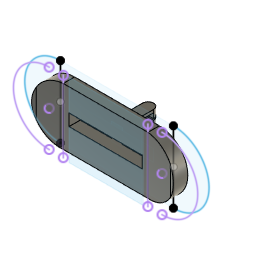
Skater v2 (Autodesk Fusion 360 design; units mm, degrees)
Autodesk Fusion 360 part; units mm, degrees
sketch "Sketch1" plane through (0, 0, 0) normal (0, 0, 1) x (1, 0, 0)
  circle A0 centre (2.87141, -3.259439) radius 3.9
  line L0 (2.87141, -3.259439) -> (6.77141, -3.259439)
  line L1 (6.77141, -3.259439) -> (-1.02859, -3.259439)
  dimension "d1" = 7.8
  constraint horizontal L0
  constraint parallel L0 L1
  measures "d1" diameter of A0
extrude "Extrude1" add sketch "Sketch1" along normal blind 3.7 contours A0 L0 L1 picked at (0.844332, -1.642898) makes body 1
sketch "Sketch2" plane through (0, 0, 0) normal (0, 0, -1) x (1, 0, 0)
  arc A0 (-1.02859, 3.259439) -> (6.77141, 3.259439) centre (2.87141, 3.259439) ccw
  line L0 (6.77141, 3.259439) -> (-1.02859, 3.259439)
  line L1 (-1.02859, 3.259439) -> (6.77141, 3.259439)
  line L2 (6.77141, 3.259439) -> (6.77141, 25.259439)
  line L3 (6.77141, 25.259439) -> (-1.02859, 25.259439)
  line L4 (-1.02859, 25.259439) -> (-1.02859, 3.259439)
  dimension "d4" = 22
  constraint horizontal L1
  constraint vertical L2
  constraint horizontal L3
  constraint vertical L4
extrude "Extrude2" add sketch "Sketch2" along normal blind 2 contours A0 L0 L1 | L0 L1 L2 L3 L4 picked at (3.53593, 1.939851) picked at (1.57141, 17.926105) bodies 1
sketch "Sketch3" plane through (6.77141, 0, 0) normal (1, 0, 0) x (0, 1, 0)
  line L0 (-3.259439, 0) -> (-25.259439, 0)
  line L1 (-25.259439, 0) -> (-25.259439, -2)
  line L2 (-25.259439, -2) -> (-3.259439, -2)
  line L3 (-3.259439, -2) -> (-3.259439, 0)
  line L4 (-12.859448, 0) -> (-15.659448, 0)
  line L5 (-14.259439, -1) -> (-12.859448, 0)
  line L6 (-14.259439, -1) -> (-15.659448, 0)
extrude "Extrude3" cut sketch "Sketch3" against normal blind 15 contours L0 L4 L5 L6 picked at (-14.259445, -0.333333) bodies 1
copy_body "CopyPasteBodies1" bodies 1 makes body 2
move_body "Move1" bodies 2 to x (1, 0, 0) y (0, 1, 0) z (0, 0, 1) at (0, 0, 6)
move_body "Move2" bodies 2 to x (-1, 0, 0) y (0, 1, 0) z (0, 0, -1) at (5.74282, 0, 14.4)
sketch "Sketch7" plane through (0, -25.259439, 0) normal (0, -1, 0) x (1, 0, 0)
  line L0 (-1.02859, 8.4) -> (6.77141, 8.4)
  line L1 (6.77141, 8.4) -> (6.77141, 10.4)
  line L2 (6.77141, 10.4) -> (-1.02859, 10.4)
  line L3 (-1.02859, 10.4) -> (-1.02859, 8.4)
sketch "Sketch8" plane through (0, 0, 10.4) normal (0, 0, 1) x (-1, 0, 0)
  line L0 (-6.77141, 25.259439) -> (-6.77141, 3.259439)
  arc A0 (-6.77141, 3.259439) -> (1.02859, 3.259439) centre (-2.87141, 3.259439) ccw
  line L1 (1.02859, 3.259439) -> (1.02859, 25.259439)
  line L2 (1.02859, 25.259439) -> (-6.77141, 25.259439)
  line L3 (-6.77141, 25.259439) -> (1.02859, 25.259439)
  line L4 (1.02859, 25.259439) -> (1.02859, 33.259439)
  line L5 (1.02859, 33.259439) -> (-6.77141, 33.259439)
  line L6 (-6.77141, 33.259439) -> (-6.77141, 25.259439)
  dimension "d10" = 8
  constraint horizontal L3
  constraint vertical L4
  constraint horizontal L5
  constraint vertical L6
sketch "Sketch9" plane through (0, 0, -2) normal (0, 0, -1) x (1, 0, 0)
  line L0 (-1.02859, 25.259439) -> (-1.02859, 3.259439)
  arc A0 (-1.02859, 3.259439) -> (6.77141, 3.259439) centre (2.87141, 3.259439) ccw
  line L1 (6.77141, 3.259439) -> (6.77141, 25.259439)
  line L2 (6.77141, 25.259439) -> (-1.02859, 25.259439)
  line L3 (-1.02859, 25.259439) -> (6.77141, 25.259439)
  line L4 (6.77141, 25.259439) -> (6.77141, 33.259439)
  line L5 (6.77141, 33.259439) -> (-1.02859, 33.259439)
  line L6 (-1.02859, 33.259439) -> (-1.02859, 25.259439)
  dimension "d11" = 8
  constraint horizontal L3
  constraint vertical L4
  constraint horizontal L5
  constraint vertical L6
extrude "Extrude4" add sketch "Sketch9" along normal blind 5 separate body contours L2 L3 L4 L5 L6 picked at (1.57141, 30.592772) makes body 3
extrude "Extrude5" add sketch "Sketch8" along normal blind 5 separate body contours L2 L3 L4 L5 L6 picked at (-4.17141, 30.592772) makes body 4
extrude "Extrude6" add 1 faces at (1.57141, -30.592772, -2) along direction (0, 0, 1) blind 2 on bodies 3 bodies 3 1
extrude "Extrude7" add 1 faces at (4.17141, -30.592772, 10.4) along direction (0, 0, -1) blind 2 on bodies 4 bodies 4 2
sketch "Sketch10" plane through (-1.02859, 0, 0) normal (-1, 0, 0) x (0, -1, 0)
  line L0 (33.259439, 8.4) -> (33.259439, 15.4)
  line L1 (33.259439, 15.4) -> (25.259439, 15.4)
  line L2 (25.259439, 15.4) -> (25.259439, 10.4)
  line L3 (25.259439, 10.4) -> (3.259439, 10.4)
  line L4 (3.259439, 10.4) -> (3.259439, 8.4)
  line L5 (3.259439, 8.4) -> (12.859448, 8.4)
  line L6 (12.859448, 8.4) -> (14.259439, 9.4)
  line L7 (14.259439, 9.4) -> (15.659448, 8.4)
  line L8 (15.659448, 8.4) -> (33.259439, 8.4)
  line L9 (12.859448, 8.4) -> (15.659448, 8.4)
sketch "Sketch11" plane through (-1.02859, 0, 0) normal (-1, 0, 0) x (0, -1, 0)
  line L0 (25.259439, -2) -> (25.259439, -7)
  line L1 (25.259439, -7) -> (33.259439, -7)
  line L2 (33.259439, -7) -> (33.259439, 0)
  line L3 (33.259439, 0) -> (15.659448, 0)
  line L4 (15.659448, 0) -> (14.259439, -1)
  line L5 (14.259439, -1) -> (12.859448, 0)
  line L6 (12.859448, 0) -> (3.259439, 0)
  line L7 (3.259439, 0) -> (3.259439, -2)
  line L8 (3.259439, -2) -> (25.259439, -2)
  line L9 (15.659448, 0) -> (12.859448, 0)
extrude "Extrude8" add sketch "Sketch10" sketch "Sketch11" against normal blind 7.8 contours L6 L7 L9 picked at (14.259445, 8.733333) of sketch 2 contours L4 L5 L9 picked at (14.259445, -0.333333) bodies 3 4
sketch "Sketch12" plane through (-1.02859, 0, 0) normal (-1, 0, 0) x (0, -1, 0)
  line L0 (33.259439, 8.4) -> (33.259439, 15.4)
  line L1 (33.259439, 15.4) -> (25.259439, 15.4)
  line L2 (25.259439, 15.4) -> (25.259439, 10.4)
  line L3 (25.259439, 10.4) -> (3.259439, 10.4)
  line L4 (3.259439, 10.4) -> (3.259439, 8.4)
  line L5 (3.259439, 8.4) -> (33.259439, 8.4)
  line L6 (25.259439, 10.4) -> (14.259439, 10.4)
  line L7 (15.659854, 10.4) -> (12.859854, 10.4)
  line L8 (12.859854, 10.4) -> (14.259439, 9.4)
  line L9 (14.259439, 9.4) -> (15.659854, 10.4)
  dimension "d23" = 2.8
extrude "Extrude9" cut sketch "Sketch12" against normal blind 8 contours L3 L6 L7 L8 L9 picked at (14.726244, 10.066667) bodies 4
sketch "Sketch13" plane through (-1.02859, 0, 0) normal (-1, 0, 0) x (0, -1, 0)
  line L0 (25.259439, -2) -> (25.259439, -7)
  line L1 (25.259439, -7) -> (33.259439, -7)
  line L2 (33.259439, -7) -> (33.259439, 0)
  line L3 (33.259439, 0) -> (3.259439, 0)
  line L4 (3.259439, 0) -> (3.259439, -2)
  line L5 (3.259439, -2) -> (25.259439, -2)
  line L6 (12.859439, -2) -> (14.259439, -1)
  line L7 (14.259439, -1) -> (15.659439, -2)
extrude "Extrude10" cut sketch "Sketch13" against normal blind 8 contours L5 L6 L7 picked at (14.259439, -1.666667) bodies 3
extrude "Extrude11" add 1 faces at (4.17141, -30.592772, 15.4) along direction (0, 0, 1) blind 15 on bodies 4 bodies 4
extrude "Extrude12" add 1 faces at (1.57141, -30.592772, -7) along direction (0, 0, -1) blind 15 on bodies 3 bodies 3
sketch "Sketch14" plane through (6.77141, 0, 0) normal (1, 0, 0) x (0, 1, 0)
  line L0 (-15.659439, -2) -> (-14.259439, -1)
  line L1 (-14.259439, -1) -> (-12.859439, -2)
  line L2 (-12.859439, -2) -> (-3.259439, -2)
  line L3 (-3.259439, -2) -> (-3.259439, 0)
  line L4 (-3.259439, 0) -> (-33.259439, 0)
  line L5 (-33.259439, 0) -> (-33.259439, -22)
  line L6 (-33.259439, -22) -> (-25.259439, -22)
  line L7 (-25.259439, -22) -> (-25.259439, -2)
  line L8 (-25.259439, -2) -> (-15.659439, -2)
  line L9 (-25.259439, -2) -> (-25.259439, 0)
  constraint perpendicular L4 L9
sketch "Sketch15" plane through (6.77141, 0, 0) normal (1, 0, 0) x (0, 1, 0)
  line L0 (-12.859854, 10.4) -> (-14.259439, 9.4)
  line L1 (-14.259439, 9.4) -> (-15.659854, 10.4)
  line L2 (-15.659854, 10.4) -> (-25.259439, 10.4)
  line L3 (-25.259439, 10.4) -> (-25.259439, 30.4)
  line L4 (-25.259439, 30.4) -> (-33.259439, 30.4)
  line L5 (-33.259439, 30.4) -> (-33.259439, 8.4)
  line L6 (-33.259439, 8.4) -> (-3.259439, 8.4)
  line L7 (-3.259439, 8.4) -> (-3.259439, 10.4)
  line L8 (-3.259439, 10.4) -> (-12.859854, 10.4)
  line L9 (-25.259439, 10.4) -> (-25.259439, 8.4)
  constraint perpendicular L6 L9
sketch "Sketch16" plane through (-1.02859, 0, 0) normal (-1, 0, 0) x (0, -1, 0)
  line L0 (15.659854, 10.4) -> (14.259439, 9.4)
  line L1 (14.259439, 9.4) -> (12.859854, 10.4)
  line L2 (12.859854, 10.4) -> (3.259439, 10.4)
  line L3 (3.259439, 10.4) -> (3.259439, 8.4)
  line L4 (3.259439, 8.4) -> (33.259439, 8.4)
  line L5 (33.259439, 8.4) -> (33.259439, 30.4)
  line L6 (33.259439, 30.4) -> (25.259439, 30.4)
  line L7 (25.259439, 30.4) -> (25.259439, 10.4)
  line L8 (25.259439, 10.4) -> (15.659854, 10.4)
  line L9 (25.259439, 10.4) -> (25.259439, 8.4)
  constraint perpendicular L4 L9
sketch "Sketch17" plane through (-1.02859, 0, 0) normal (-1, 0, 0) x (0, -1, 0)
  line L0 (14.259439, -1) -> (15.659439, -2)
  line L1 (15.659439, -2) -> (25.259439, -2)
  line L2 (25.259439, -2) -> (25.259439, -22)
  line L3 (25.259439, -22) -> (33.259439, -22)
  line L4 (33.259439, -22) -> (33.259439, 0)
  line L5 (33.259439, 0) -> (3.259439, 0)
  line L6 (3.259439, 0) -> (3.259439, -2)
  line L7 (3.259439, -2) -> (12.859439, -2)
  line L8 (12.859439, -2) -> (14.259439, -1)
  line L9 (25.259439, -2) -> (25.259439, 0)
  constraint perpendicular L5 L9
extrude "Extrude13" add sketch "Sketch17" sketch "Sketch16" along normal blind 7 contours L2 L3 L4 L5 L9 picked at (30.592772, -8) of sketch 2 contours L4 L5 L6 L7 L9 picked at (30.592772, 16.4) bodies 3 4
extrude "Extrude14" add sketch "Sketch15" sketch "Sketch14" along normal blind 7 contours L3 L4 L5 L6 L9 picked at (-30.592772, 16.4) of sketch 2 contours L4 L5 L6 L7 L9 picked at (-30.592772, -8) bodies 3 4
extrude "Extrude15" add 2 faces at (-8.02859, -30.592772, 23.066667) (-8.02859, -27.926105, -7.333333) along direction (-1, 0, 0) blind 15 on bodies 3 4 bodies 4 3
extrude "Extrude16" add 2 faces at (13.77141, -27.926105, 15.733333) (13.77141, -27.926105, -14.666667) along direction (1, 0, 0) blind 15 on bodies 3 4 bodies 4 3
sketch "Sketch18" plane through (0, -33.259439, 0) normal (0, -1, 0) x (1, 0, 0)
  line L0 (-23.02859, -22) -> (28.77141, -22)
  line L1 (28.77141, -22) -> (28.77141, 0)
  line L2 (28.77141, 0) -> (-23.02859, 0)
  line L3 (-23.02859, 0) -> (-23.02859, -22)
sketch "Sketch19" plane through (0, -33.259439, 0) normal (0, -1, 0) x (1, 0, 0)
  line L0 (28.77141, 30.4) -> (-23.02859, 30.4)
  line L1 (-23.02859, 30.4) -> (-23.02859, 8.4)
  line L2 (-23.02859, 8.4) -> (28.77141, 8.4)
  line L3 (28.77141, 8.4) -> (28.77141, 30.4)
sketch "Sketch20" plane through (28.77141, 0, 0) normal (1, 0, 0) x (0, 1, 0)
  line L0 (-25.259439, 30.4) -> (-33.259439, 30.4)
  line L1 (-33.259439, 30.4) -> (-33.259439, 8.4)
  line L2 (-33.259439, 8.4) -> (-25.259439, 8.4)
  line L3 (-25.259439, 8.4) -> (-25.259439, 30.4)
  line L4 (-33.259439, 30.4) -> (-25.259439, 30.4)
  line L5 (-25.259439, 30.4) -> (-25.259439, 1.557933)
  line L6 (-25.259439, 1.557933) -> (-33.259439, 1.557933)
  line L7 (-33.259439, 1.557933) -> (-33.259439, 30.4)
  constraint horizontal L4
  constraint vertical L5
  constraint horizontal L6
  constraint vertical L7
sketch "Sketch21" plane through (28.77141, 0, 0) normal (1, 0, 0) x (0, 1, 0)
  line L0 (-25.259439, -22) -> (-25.259439, 0)
  line L1 (-25.259439, 0) -> (-33.259439, 0)
  line L2 (-33.259439, 0) -> (-33.259439, -22)
  line L3 (-33.259439, -22) -> (-25.259439, -22)
  line L4 (-25.259439, -22) -> (-33.259439, -22)
  line L5 (-33.259439, -22) -> (-33.259439, 7.010698)
  line L6 (-33.259439, 7.010698) -> (-25.259439, 7.010698)
  line L7 (-25.259439, 7.010698) -> (-25.259439, -22)
  constraint horizontal L4
  constraint vertical L5
  constraint horizontal L6
  constraint vertical L7
extrude "Extrude17" add sketch "Sketch20" sketch "Sketch21" along normal blind 1 contours L0 L1 L2 L3 L4 L5 L7 | L2 L5 L6 L7 picked at (-27.926105, 15.733333) picked at (-30.592772, 6.119311) of sketch 2 contours L0 L1 L2 L3 L4 L5 L7 | L1 L5 L6 L7 picked at (-27.926105, -14.666667) picked at (-30.592772, 4.673798) bodies 3 4
sketch "Sketch22" plane through (0, -33.259439, 0) normal (0, -1, 0) x (1, 0, 0)
sketch "Sketch23" plane through (2.87141, -33.259439, -11) normal (0, -1, 0) x (1, 0, 0)
sketch "Sketch24" plane through (0, -33.259439, 0) normal (0, -1, 0) x (1, 0, 0)
sketch "Sketch25" plane through (0, -33.259439, 0) normal (0, -1, 0) x (1, 0, 0)
  line L0 (-23.02859, -22) -> (29.77141, -22)
  line L1 (29.77141, -22) -> (29.77141, 30.4)
  line L2 (29.77141, 30.4) -> (-23.02859, 30.4)
  line L3 (-23.02859, 30.4) -> (-23.02859, 8.4)
  line L4 (-23.02859, 8.4) -> (28.77141, 8.4)
  line L5 (28.77141, 8.4) -> (28.77141, 0)
  line L6 (28.77141, 0) -> (-23.02859, 0)
  line L7 (-23.02859, 0) -> (-23.02859, -22)
extrude "Extrude18" add 1 faces at (29.77141, -30.592772, 12.933333) along direction (1, 0, 0) blind 13 on bodies 3 bodies 3
sketch "Sketch26" plane through (-23.02859, 0, 0) normal (-1, 0, 0) x (0, -1, 0)
  line L0 (25.259439, 30.4) -> (25.259439, 8.4)
  line L1 (25.259439, 8.4) -> (33.259439, 8.4)
  line L2 (33.259439, 8.4) -> (33.259439, 30.4)
  line L3 (33.259439, 30.4) -> (25.259439, 30.4)
  line L4 (25.259439, 30.4) -> (33.259439, 30.4)
  line L5 (33.259439, 30.4) -> (33.259439, -16.961033)
  line L6 (33.259439, -16.961033) -> (25.259439, -16.961033)
  line L7 (25.259439, -16.961033) -> (25.259439, 30.4)
  constraint horizontal L4
  constraint vertical L5
  constraint horizontal L6
  constraint vertical L7
sketch "Sketch27" plane through (-23.02859, 0, 0) normal (-1, 0, 0) x (0, -1, 0)
  line L0 (25.259439, -22) -> (33.259439, -22)
  line L1 (33.259439, -22) -> (33.259439, 0)
  line L2 (33.259439, 0) -> (25.259439, 0)
  line L3 (25.259439, 0) -> (25.259439, -22)
  line L4 (33.259439, -22) -> (25.259439, -22)
  line L5 (25.259439, -22) -> (25.259439, -5.279262)
  line L6 (25.259439, -5.279262) -> (33.259439, -5.279262)
  line L7 (33.259439, -5.279262) -> (33.259439, -22)
  constraint horizontal L4
  constraint vertical L5
  constraint horizontal L6
  constraint vertical L7
extrude "Extrude19" add sketch "Sketch26" sketch "Sketch27" along normal blind 14 contours L0 L1 L2 L3 L4 L5 L7 | L1 L5 L6 L7 picked at (27.926105, 23.066667) picked at (30.592772, -8.507356) of sketch 2 contours L0 L1 L3 L4 L5 L6 L7 picked at (27.926105, -10.852841) bodies 3
sketch "Sketch28" plane through (0, -33.259439, 0) normal (0, -1, 0) x (1, 0, 0)
  line L0 (-23.02859, 8.4) -> (28.77141, 8.4)
  line L1 (28.77141, 8.4) -> (28.77141, 0)
  line L2 (28.77141, 0) -> (-23.02859, 0)
  line L3 (-23.02859, 0) -> (-23.02859, 8.4)
  line L4 (42.77141, 30.4) -> (-37.02859, 30.4)
  line L5 (-37.02859, 30.4) -> (-37.02859, -22)
  line L6 (-37.02859, -22) -> (42.77141, -22)
  line L7 (42.77141, -22) -> (42.77141, 30.4)
  arc A0 (-37.02859, 30.4) -> (-37.02859, -22) centre (-37.02859, 4.2) ccw
  arc A1 (42.77141, -22) -> (42.77141, 30.4) centre (42.77141, 4.2) ccw
  constraint tangent L6 A0
  constraint tangent L4 A0
  constraint tangent L6 A1
  constraint tangent L4 A1
extrude "Extrude20" add sketch "Sketch28" against normal blind 8 contours L7 A1 | L5 A0 picked at (51.480323, 4.852643) picked at (-45.737503, 3.547357) bodies 3
extrude "Extrude21" add 1 faces at (11.504743, -33.259439, -14.666667) along direction (0, -1, 0) blind 5 thin wall 1 inside on bodies 3 bodies 3
sketch "Sketch29" plane through (0, -33.259439, 0) normal (0, -1, 0) x (1, 0, 0)
  line L0 (-24.02859, -1) -> (-24.02859, 9.4)
  line L1 (-24.02859, 9.4) -> (29.77141, 9.4)
  line L2 (29.77141, 9.4) -> (29.77141, -1)
  line L3 (29.77141, -1) -> (-24.02859, -1)
  line L4 (42.77141, 29.4) -> (-37.02859, 29.4)
  arc A0 (-37.02859, 29.4) -> (-37.02859, -21) centre (-37.02859, 4.2) ccw
  line L5 (-37.02859, -21) -> (42.77141, -21)
  arc A1 (42.77141, -21) -> (42.77141, 29.4) centre (42.77141, 4.2) ccw
  line L6 (-37.02859, 29.4) -> (-27.02859, 29.4)
  line L7 (42.77141, 29.4) -> (32.77141, 29.4)
  line L8 (32.77141, 29.4) -> (32.77141, -21)
  line L9 (-27.02859, 29.4) -> (-27.02859, -21)
  dimension "d55" = 10
  dimension "d56" = 10
  constraint perpendicular L0 L6
  constraint parallel L4 L7
  constraint perpendicular L5 L8
  constraint perpendicular L5 L9
sketch "Sketch30" plane through (0, -33.259439, 0) normal (0, -1, 0) x (1, 0, 0)
sketch "Sketch31" plane through (0, -33.259439, 0) normal (0, -1, 0) x (1, 0, 0)
sketch "Sketch32" plane through (0, -33.259439, 0) normal (0, -1, 0) x (1, 0, 0)
sketch "Sketch33" plane through (0, 0, 0) normal (0, 1, 0) x (1, 0, 0)
sketch "Sketch35" plane through (-44.62859, -33.259439, 4.2) normal (0, -1, 0) x (1, 0, 0)
  line L0 (17.6, 25.2) -> (17.6, -25.2)
  arc A0 (7.6, 25.2) -> (7.6, -25.2) centre (7.6, 0) ccw
  line L1 (77.4, 25.2) -> (77.4, -25.2)
  arc A1 (87.4, -25.2) -> (87.4, 25.2) centre (87.4, 0) ccw
revolve "Revolve1" add sketch "Sketch29" angle 5 about axis through (-27.02859, -33.259439, 29.4) along (0, 0, 1) contours L4 A0 L5 L6 L9 picked at (-42.742041, -1.957636) bodies 3
sketch "Sketch36" plane through (0, -33.259439, 0) normal (0, -1, 0) x (1, 0, 0)
  line L0 (-27.02859, 29.4) -> (-27.02859, -21)
  line L1 (-27.02859, -21) -> (42.77141, -21)
  arc A0 (42.77141, -21) -> (42.77141, 29.4) centre (42.77141, 4.2) ccw
  line L2 (42.77141, 29.4) -> (-27.02859, 29.4)
  line L3 (-24.02859, -1) -> (-24.02859, 9.4)
  line L4 (-24.02859, 9.4) -> (29.77141, 9.4)
  line L5 (29.77141, 9.4) -> (29.77141, -1)
  line L6 (29.77141, -1) -> (-24.02859, -1)
  line L7 (32.77141, 29.4) -> (32.77141, -21)
  point P0 (32.77141, 29.4)
  point P1 (32.77141, -21)
revolve "Revolve2" add sketch "Sketch36" angle 5 about axis through (32.77141, -33.259439, 29.4) along (0, 0, -1) contours L1 A0 L2 L7 picked at (54.605428, 5.237314) bodies 3
sketch "Sketch37" plane through (-2.638785, -30.161448, 0) normal (-0.087156, -0.996195, 0) x (0.996195, -0.087156, 0)
  line L0 (35.545456, 29.4) -> (35.545456, -21)
  line L1 (35.545456, -21) -> (45.545456, -21)
  arc A0 (45.545456, -21) -> (45.545456, 29.4) centre (45.545456, 4.2) ccw
  line L2 (45.545456, 29.4) -> (35.545456, 29.4)
  line L3 (53.145456, -19.826652) -> (53.145456, 28.226652)
sketch "Sketch38" plane through (2.682408, -30.660063, 0) normal (0.087156, -0.996195, 0) x (0.996195, 0.087156, 0)
  arc A0 (-39.824489, 29.4) -> (-39.824489, -21) centre (-39.824489, 4.2) ccw
  line L0 (-39.824489, -21) -> (-29.824489, -21)
  line L1 (-29.824489, -21) -> (-29.824489, 29.4)
  line L2 (-29.824489, 29.4) -> (-39.824489, 29.4)
  line L3 (-47.424489, 28.226652) -> (-47.424489, -19.826652)
revolve "Revolve3" add sketch "Sketch37" angle 10 about axis through (50.304437, -34.79338, -19.826652) along (0, 0, -1) contours A0 L3 picked at (57.899083, 0.021459) bodies 3
revolve "Revolve4" add sketch "Sketch38" angle 10 about axis through (-44.561617, -34.79338, 28.226652) along (0, 0, 1) contours A0 L3 picked at (-56.476506, 1.698018) bodies 3
sketch "Sketch39" plane through (-5.328587, -19.886556, 0) normal (-0.258819, -0.965926, 0) x (0.965926, -0.258819, 0)
  arc A0 (57.595544, -19.826652) -> (57.595544, 28.226652) centre (49.995544, 4.2) ccw
  line L0 (57.595544, 28.226652) -> (57.595544, -19.826652)
  line L1 (66.395544, -14.933217) -> (66.395544, 23.333217)
sketch "Sketch40" plane through (5.713283, -21.322261, 0) normal (0.258819, -0.965926, 0) x (0.965926, 0.258819, 0)
  arc A0 (-52.048406, 28.226652) -> (-52.048406, -19.826652) centre (-44.448406, 4.2) ccw
  line L0 (-52.048406, -19.826652) -> (-52.048406, 28.226652)
  line L1 (-60.848406, -14.933217) -> (-60.848406, 23.333217)
revolve "Revolve5" add sketch "Sketch40" angle 10 about axis through (-53.061764, -37.070987, -14.933217) along (0, 0, 1) contours A0 L1 picked at (-64.55212, 2.148555) bodies 3
revolve "Revolve6" add sketch "Sketch39" angle 10 about axis through (58.804584, -37.070987, -14.933217) along (0, 0, -1) contours A0 L1 picked at (67.979106, 8.766647) bodies 3
extrude "Extrude22" cut 1 faces at (-10.42859, -38.259439, -21.333333) along direction (0, 1, 0) blind 20 on bodies 3 bodies 3
extrude "Extrude23" cut 1 faces at (-5.761923, -38.259439, -0.666667) along direction (0, 1, 0) blind 5 on bodies 3 bodies 3
sketch "Sketch41" plane through (0, -25.259439, 0) normal (0, 1, 0) x (-1, 0, 0)
  line L0 (-42.77141, -21) -> (37.02859, -21)
  arc A0 (37.02859, -21) -> (37.02859, 29.4) centre (37.02859, 4.2) ccw
  line L1 (37.02859, 29.4) -> (-42.77141, 29.4)
  arc A1 (-42.77141, 29.4) -> (-42.77141, -21) centre (-42.77141, 4.2) ccw
  line L2 (23.02859, 8.4) -> (23.02859, 0)
  line L3 (23.02859, 0) -> (1.02859, 0)
  line L4 (1.02859, 0) -> (1.02859, -2)
  line L5 (1.02859, -2) -> (-6.77141, -2)
  line L6 (-6.77141, -2) -> (-6.77141, 0)
  line L7 (-6.77141, 0) -> (-28.77141, 0)
  line L8 (-28.77141, 0) -> (-28.77141, 8.4)
  line L9 (-28.77141, 8.4) -> (-6.77141, 8.4)
  line L10 (-6.77141, 8.4) -> (-6.77141, 10.4)
  line L11 (-6.77141, 10.4) -> (1.02859, 10.4)
  line L12 (1.02859, 10.4) -> (1.02859, 8.4)
  line L13 (1.02859, 8.4) -> (23.02859, 8.4)
  line L14 (-42.77141, 29.4) -> (-42.77141, -21)
  line L15 (37.02859, -21) -> (37.02859, 29.4)
sketch "Sketch42" plane through (0, -25.259439, 0) normal (0, 1, 0) x (-1, 0, 0)
  arc A0 (-42.77141, 29.4) -> (-42.77141, -21) centre (-42.77141, 4.2) ccw
  arc A1 (37.02859, -21) -> (37.02859, 29.4) centre (37.02859, 4.2) ccw
  point P0 (-42.77141, 29.4)
  point P1 (-42.77141, -21)
  point P2 (37.02859, -21)
  point P3 (37.02859, 29.4)
chamfer "Chamfer1" distance 5 angle 45 4 edges at (67.97141, -25.259439, 4.2) (2.87141, -25.259439, -21) (-62.22859, -25.259439, 4.2) (2.87141, -25.259439, 29.4) on bodies 3
sketch "Sketch43" plane through (6.77141, 0, 0) normal (1, 0, 0) x (0, 1, 0)
  line L0 (-25.259439, 10.4) -> (-25.259439, 8.4)
  line L1 (-25.259439, 8.4) -> (-3.259439, 8.4)
  line L2 (-3.259439, 8.4) -> (-3.259439, 10.4)
  line L3 (-3.259439, 10.4) -> (-12.859854, 10.4)
  line L4 (-12.859854, 10.4) -> (-14.259439, 9.4)
  line L5 (-14.259439, 9.4) -> (-15.659854, 10.4)
  line L6 (-15.659854, 10.4) -> (-25.259439, 10.4)
  line L7 (-12.859854, 10.4) -> (-15.659854, 10.4)
  line L8 (-15.659854, 10.4) -> (-15.659854, 8.4)
  line L9 (-12.859854, 10.4) -> (-12.859854, 8.4)
  line L10 (-12.859854, 8.4) -> (-14.259439, 9.4)
  line L11 (-14.259439, 9.4) -> (-15.659854, 8.4)
  constraint perpendicular L1 L8
  constraint perpendicular L1 L9
sketch "Sketch44" plane through (6.77141, 0, 0) normal (1, 0, 0) x (0, 1, 0)
  line L0 (-25.259439, 0) -> (-25.259439, -2)
  line L1 (-25.259439, -2) -> (-15.659439, -2)
  line L2 (-15.659439, -2) -> (-14.259439, -1)
  line L3 (-14.259439, -1) -> (-12.859439, -2)
  line L4 (-12.859439, -2) -> (-3.259439, -2)
  line L5 (-3.259439, -2) -> (-3.259439, 0)
  line L6 (-3.259439, 0) -> (-25.259439, 0)
  line L7 (-12.859439, -2) -> (-12.859439, 0)
  line L8 (-12.859439, 0) -> (-14.259439, -1)
  line L9 (-15.659439, -2) -> (-15.659439, 0)
  line L10 (-14.259439, -1) -> (-15.659439, 0)
  line L11 (-12.859439, -2) -> (-13.063744, -2)
  line L12 (-13.063744, -2) -> (-15.659439, -2)
  constraint perpendicular L6 L7
  constraint perpendicular L6 L9
  constraint perpendicular L7 L11
  constraint perpendicular L9 L12
extrude "Extrude24" cut sketch "Sketch43" sketch "Sketch44" against normal blind 8 contours L4 L5 L7 | L1 L10 L11 picked at (-14.259715, 10.066667) picked at (-14.259715, 8.733333) of sketch 2 contours L6 L8 L10 | L2 L3 L11 L12 picked at (-14.259439, -0.333333) picked at (-14.327541, -1.666667) bodies 3
sketch "Sketch45" plane through (-1.02859, 0, 0) normal (-1, 0, 0) x (0, -1, 0)
  line L0 (14.259439, -1) -> (12.859439, 0)
  line L1 (12.859439, 0) -> (3.259439, 0)
  line L2 (3.259439, 0) -> (3.259439, -2)
  line L3 (3.259439, -2) -> (12.859439, -2)
  line L4 (12.859439, -2) -> (14.259439, -1)
  line L5 (12.859439, -2) -> (14.259439, -1)
  line L6 (15.659439, -2) -> (12.859439, -2)
  line L7 (14.259439, -1) -> (15.659439, -2)
  constraint parallel L3 L6
  constraint parallel L0 L7
sketch "Sketch46" plane through (-1.02859, 0, 0) normal (-1, 0, 0) x (0, -1, 0)
  line L0 (12.859854, 8.4) -> (14.259439, 9.4)
  line L1 (14.259439, 9.4) -> (12.859854, 10.4)
  line L2 (12.859854, 10.4) -> (3.259439, 10.4)
  line L3 (3.259439, 10.4) -> (3.259439, 8.4)
  line L4 (3.259439, 8.4) -> (12.859854, 8.4)
  line L5 (12.859854, 10.4) -> (14.259439, 9.4)
  line L6 (14.259439, 10.4) -> (12.859854, 10.4)
  line L7 (12.859854, 10.4) -> (15.659854, 10.4)
  line L8 (14.259439, 9.4) -> (15.659854, 10.4)
  dimension "d70" = 2.8
  constraint parallel L6 L7
sketch "Sketch47" plane through (-1.02859, -14.259854, 9.9) normal (-1, 0, 0) x (0, -1, 0)
extrude "Extrude25" add sketch "Sketch45" sketch "Sketch46" against normal blind 7.8 contours L4 L5 L6 L7 picked at (14.259439, -1.666667) of sketch 2 contours L1 L5 L6 L7 L8 picked at (14.726244, 10.066667) bodies 3
sketch "Sketch48" plane through (3.37141, -33.259439, 4.2) normal (0, -1, 0) x (1, 0, 0)
  line L0 (-30.4, 25.2) -> (-30.4, 20.2)
  line L1 (29.4, 25.2) -> (29.4, 20.2)
  line L2 (-30.4, 20.2) -> (29.4, 20.2)
  line L3 (-30.4, 20.2) -> (29.4, 20.2)
  line L4 (29.4, 20.2) -> (29.4, -20.2)
  line L5 (29.4, -20.2) -> (-30.4, -20.2)
  line L6 (-30.4, -20.2) -> (-30.4, 20.2)
  arc A0 (-30.4, 20.2) -> (-30.4, -20.2) centre (-30.4, 0) ccw
  arc A1 (29.4, -20.2) -> (29.4, 20.2) centre (29.4, 0) ccw
  arc A2 (-40.4, 25.2) -> (-40.4, -25.2) centre (-45.400922, 0) ccw
  arc A3 (-40.4, 25.2) -> (-40.4, -25.2) centre (-40.4, 0) ccw
  arc A4 (39.4, -25.2) -> (39.4, 25.2) centre (45.182249, 0) ccw
  line L7 (-40.4, 25.2) -> (39.4, 25.2)
  line L8 (39.4, -25.2) -> (-40.4, -25.2)
  point P0 (-30.4, 25.2)
  point P1 (29.4, 25.2)
  point P2 (39.4, -25.2)
  dimension "d73" = 5
  dimension "d74" = 5
  dimension "d75" = 40.4
  constraint coincident P0 L0.start
  constraint coincident P1 L1.start
  constraint perpendicular L1 L2
  constraint horizontal L3
  constraint vertical L4
  constraint horizontal L5
  constraint vertical L6
  constraint tangent L5 A0
  constraint coincident A2.end A3
  constraint coincident A2.start A3
  constraint coincident P2 A4.start
  constraint tangent A3 L7
  constraint tangent A3 L8
  measures "d73" distance of P0 L0.end
  measures "d74" distance of P1 L1.end
  measures "d75" distance of L0.end L5.end
extrude "Extrude26" add sketch "Sketch48" along normal blind 28 contours L0 L1 L2 L3 L7 | L0 L1 L5 A0 A1 A3 A4 L7 L8 picked at (-10.466667, 23.533333) picked at (-10.466667, -23.533333) bodies 3
extrude "Extrude27" cut 1 faces at (12.838077, -61.259439, 27.733333) along direction (0, 1, 0) blind 75 on bodies 3 bodies 3
